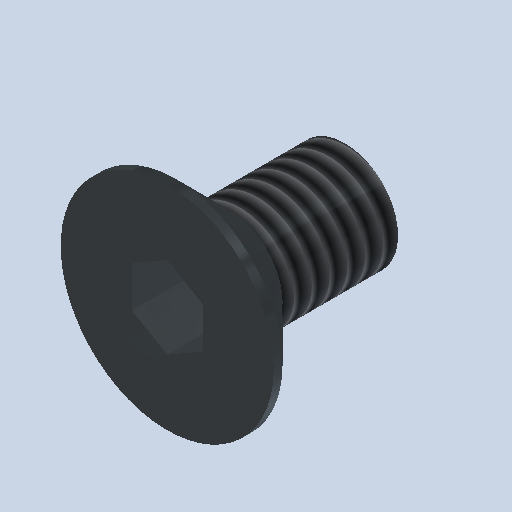
# Autodesk Inventor part: m3皿ネジ5 (1)
Saved by Autodesk Inventor 2022 (Build 260153000, 153)
## iProperties
Created: 2015-01-12
Part Number: m3皿ネジ5 (1)
Material: 鉄 灰色
Document SubType Name: Modeling
Designer: Riku
Density: 7.15 g/cm^3
Appearance: 鉄 灰色
Mass: 0.354535 g
Surface Area: 1.11068 cm^2
Volume: 0.0495854 cm^3
Author: Riku
Autodesk Inventor part; units mm, degrees
ref_plane "YZ Plane" through (0, 0, 0) normal (1, 0, 0) x (0, 1, 0)
ref_plane "XZ Plane" through (0, 0, 0) normal (0, 1, 0) x (-1, 0, 0)
ref_plane "XY Plane" through (0, 0, 0) normal (0, 0, 1) x (1, 0, 0)
sketch "スケッチ1" plane through (0, 0, 0) normal (0, 0, 1) x (1, 0, 0)
  circle A0 centre (0, 0) radius 1.5
  dimension "d0" = 3
  constraints: 1 centre point, 1 coincident
  measures "d0" diameter of A0
extrude "押し出し1" add sketch "スケッチ1" along normal blind 5
thread "ねじ1" size "M3x0.5" class "6g" standard "ANSI Metric M Profile" full length
sketch "スケッチ2" plane through (0, 0, 5) normal (0, 0, 1) x (1, 0, 0)
  circle A0 centre (0, 0) radius 3
  dimension "d5" = 6
  constraints: 1 centre point, 1 coincident
  measures "d5" diameter of A0
extrude "押し出し2" add sketch "スケッチ2" against normal blind 1.75
chamfer "面取り1" distance 1.5 angle 45 1 edges at (-3, 0, 3.25)
sketch "スケッチ3" plane through (0, 0, 5) normal (0, 0, 1) x (1, 0, 0)
  line L0 (0, 1.1547) -> (1, 0.5774)
  line L1 (1, 0.5774) -> (1, -0.5774)
  line L2 (1, -0.5774) -> (0, -1.1547)
  line L3 (0, -1.1547) -> (-1, -0.5774)
  line L4 (-1, -0.5774) -> (-1, 0.5774)
  line L5 (-1, 0.5774) -> (0, 1.1547)
  point P0 (0, 0)
  point P1 (0, 0)
  dimension "d11" = 2
  constraints: 12 end point, 1 coincident, 13 other
  measures "d11" distance between parallel lines of L1 L4
extrude "押し出し3" cut sketch "スケッチ3" against normal blind 1.5
